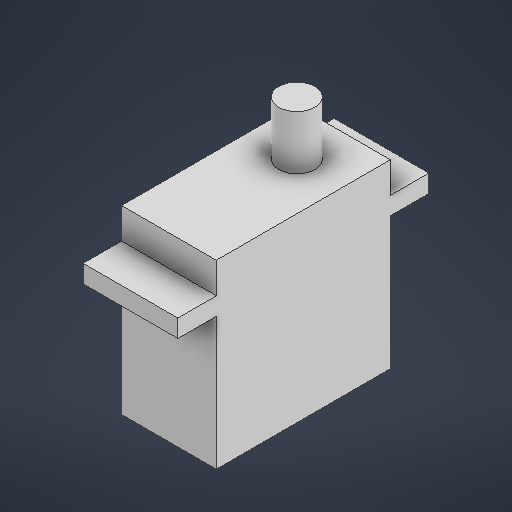
# Autodesk Inventor part: testingservo
Saved by Autodesk Inventor 2026.2 (Build 302298000, 298)
## iProperties
Created: 2026-04-07
Part Number: testingservo
Material: Generic
Document SubType Name: Modeling
Designer: Brian Wang
Density: 1 g/cm^3
Appearance: Default
Author: Brian Wang
Autodesk Inventor part; units mm, degrees
ref_plane "YZ Plane" through (0, 0, 0) normal (1, 0, 0) x (0, 1, 0)
ref_plane "XZ Plane" through (0, 0, 0) normal (0, 1, 0) x (-1, 0, 0)
ref_plane "XY Plane" through (0, 0, 0) normal (0, 0, 1) x (1, 0, 0)
sketch "Sketch1" plane through (0, 0, 0) normal (0, 1, 0) x (-1, 0, 0)
  line L0 (-17.8956, 13.1221) -> (-17.8956, -9.4779)
  line L1 (-17.8956, -9.4779) -> (-5.5956, -9.4779)
  line L2 (-5.5956, -9.4779) -> (-5.5956, 13.1221)
  line L3 (-5.5956, 13.1221) -> (-17.8956, 13.1221)
  point P0 (0, 0)
  dimension "d0" = 22.6
  dimension "d1" = 12.3
  constraints: 8 end point, 2 parallel, 1 perpendicular
  measures "d0" distance of L2.end L1.end
  measures "d1" distance of L1.end L0.end
extrude "Extrusion1" add sketch "Sketch1" along normal blind 23.5
sketch "Sketch2" plane through (17.8956, 0, -9.4779) normal (0, 0, -1) x (-1, 0, 0)
  line L0 (0, 0) -> (0, 23.5) projected
  line L1 (12.3, 0) -> (12.3, 23.5) projected
  line L2 (0, 17.2) -> (12.3, 17.2)
  line L3 (12.3, 17.2) -> (12.3, 19.5)
  line L4 (12.3, 19.5) -> (0, 19.5)
  line L5 (0, 19.5) -> (0, 17.2)
  line L6 (0, 0) -> (12.3, 0) projected
  point P0 (17.8956, 0)
  point P1 (0, 19.5)
  dimension "d4" = 17.2
  dimension "d5" = 2.3
  constraints: 8 end point, 2 parallel, 2 point on line, 1 horizontal, 1 perpendicular
  measures "d4" distance between parallel lines of L6 L2
  measures "d5" distance between parallel lines of L2 L4
extrude "Extrusion2" add sketch "Sketch2" along normal blind 5 contours L0 L4 L1 L2
sketch "Sketch3" plane through (5.5956, 0, 13.1221) normal (0, 0, 1) x (1, 0, 0)
  line L0 (0, 19.5) -> (12.3, 19.5) projected
  line L1 (12.3, 17.2) -> (0, 17.2) projected
  line L2 (12.3, 19.5) -> (0, 19.5)
  line L3 (0, 19.5) -> (0, 17.2)
  line L4 (0, 17.2) -> (12.3, 17.2)
  line L5 (12.3, 17.2) -> (12.3, 19.5)
  point P0 (-5.5956, 0)
  point P1 (0, 19.5)
  point P2 (12.3, 17.2)
  constraints: 8 end point, 2 parallel, 1 horizontal, 1 perpendicular
extrude "Extrusion3" add sketch "Sketch3" along normal blind 5
sketch "Sketch4" plane through (0, 23.5, 0) normal (0, 1, 0) x (1, 0, 0)
  circle A0 centre (11.7456, 3.4779) radius 2.35
  line L0 (17.8956, 9.4779) -> (5.5956, 9.4779) projected
  point P0 (0, 0)
  dimension "d10" = 4.7
  dimension "d11" = 6
  constraints: 1 centre point
  measures "d10" diameter of A0
  measures "d11" distance from line of L0 A0.centre
extrude "Extrusion4" add sketch "Sketch4" along normal blind 7
body "Solid1"
